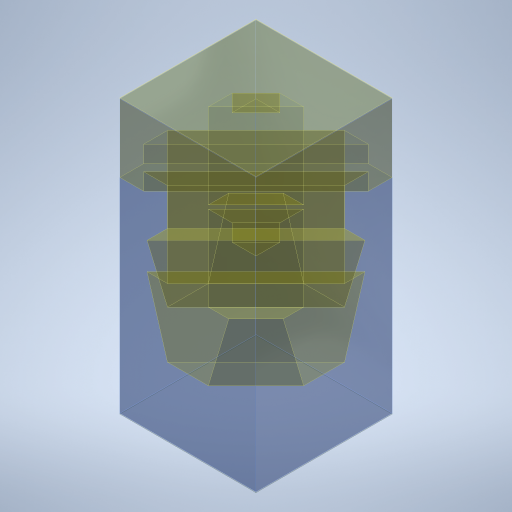
# Autodesk Inventor part: J1
Saved by Autodesk Inventor 2024 (Build 280153000, 153)
## iProperties
Created: 2013-03-22
Part Number: J1
Material: Generic
Document SubType Name: Modeling
Designer: User
Density: 1 g/cm^3
Appearance: Default
Author: User
Autodesk Inventor part; units mm, degrees
ref_plane "YZ Plane" through (0, 0, 0) normal (1, 0, 0) x (0, 1, 0)
ref_plane "XY Plane" through (0, 0, 0) normal (0, 0, 1) x (1, 0, 0)
ref_plane "Work Plane1" through (0, 180, -120) normal (0, 1, 0) x (-1, 0, 0)
sketch "Sketch3" plane through (0, 0, 0) normal (0, 0, 1) x (1, 0, 0)
  line L0 (-36, 180) -> (216, 180) projected
  line L1 (0, 0) -> (180, 0)
  line L2 (180, 0) -> (180, 180)
  line L3 (180, 180) -> (0, 180)
  line L4 (0, 180) -> (0, 0)
  dimension "d3" = 180
  constraints: 8 end point, 2 parallel, 2 perpendicular, 1 collinear, 1 horizontal
  measures "d3" distance of L3.end L1.start
extrude "Extrusion1" add sketch "Sketch3" along normal blind 360
ref_plane "Midlle" through (180, 180, 180) normal (0, 0, 1) x (1, 0, 0)
ref_plane "Work Plane2" through (180, 0, 0) normal (-0.7071068, -0.7071068, 0) x (0, 0, 1)
sketch "Sketch4" plane through (180, 0, 0) normal (-0.7071068, -0.7071068, 0) x (0, 0, 1)
  line L0 (360, 0) -> (0, 0) projected
  line L1 (0, 0) -> (0, 254.5584) projected
  line L2 (0, 254.5584) -> (360, 254.5584) projected
  line L3 (360, 254.5584) -> (360, 0) projected
  line L4 (0, 127.2792) -> (360, 127.2792) construction
  line L5 (270, 254.5584) -> (270, 232.2846)
  line L6 (270, 232.2846) -> (292.2739, 232.2846)
  line L7 (292.2739, 232.2846) -> (292.2739, 210.0107)
  line L8 (292.2739, 210.0107) -> (180, 210.0107)
  line L9 (180, 210.0107) -> (180, 229.1026)
  line L10 (180, 229.1026) -> (90, 210.0107)
  line L11 (90, 210.0107) -> (90, 171.8269)
  line L12 (90, 171.8269) -> (180, 152.7351)
  line L13 (180, 152.7351) -> (180, 171.8269)
  line L14 (180, 171.8269) -> (292.2739, 171.8269)
  line L15 (292.2739, 171.8269) -> (292.2739, 82.7315)
  line L16 (34.5859, 254.5584) -> (34.5859, 127.2792) construction
  line L17 (34.5859, 190.9188) -> (15.3416, 190.9188) construction
  line L18 (270, 22.2739) -> (292.2739, 22.2739)
  line L19 (292.2739, 22.2739) -> (292.2739, 44.5477)
  line L20 (292.2739, 44.5477) -> (180, 44.5477)
  line L21 (180, 44.5477) -> (180, 25.4558)
  line L22 (180, 25.4558) -> (90, 44.5477)
  line L23 (90, 44.5477) -> (90, 82.7315)
  line L24 (90, 82.7315) -> (180, 101.8234)
  line L25 (180, 101.8234) -> (180, 82.7315)
  line L26 (180, 82.7315) -> (292.2739, 82.7315)
  line L27 (270, 22.2739) -> (270, 0)
  line L28 (292.2739, 105.0054) -> (270, 105.0054)
  line L29 (270, 105.0054) -> (270, 149.5531)
  line L30 (270, 149.5531) -> (292.2739, 149.5531)
  line L31 (292.2739, 149.5531) -> (292.2739, 105.0054)
  line L32 (281.1369, 105.0054) -> (281.1369, 127.2792) construction
  point P0 (292.2739, 127.2792)
  dimension "d6" = 254.5584
  dimension "d9" = 360
  dimension "d25" = 127.2792
  dimension "d26" = 76.3675
  dimension "d27" = 19.0919
  dimension "d28" = 90
  dimension "d29" = 90
  dimension "d30" = 90
  constraints: 56 end point, 10 symmetric about line, 9 parallel, 7 perpendicular, 7 point on line, 4 midpoint, 3 equal length, 2 collinear, 1 horizontal, 3 other
  measures "d6" distance of L0.end L1.end
  measures "d9" distance of L1.end L2.end
  measures "d25" distance between parallel lines of L2 L4
  measures "d26" distance of L12.end L9.end
  measures "d27" distance of L8.end L9.end
  measures "d28" distance between parallel lines of L1 L11
  measures "d29" distance between parallel lines of L9 L11
  measures "d30" distance between parallel lines of L3 L5
extrude "Extrusion7" add sketch "Sketch4" against normal up to surface separate body contours L0 L27 L18 L19 L20 L21 L22 L23 L24 L25 L26 L15 L14 L13 L12 L11 L10 L9 L8 L7 L6 L5 L2 L3 | L28 L29 L30 L15 starts on plane at (0, 0, 0) facing (0, -1, 0) surface through (180, 180, 0) normal (0, 1, 0)
extrude "Extrusion8" cut sketch "Sketch3" along normal blind 360 keep common part bodies 2
extrude "Extrusion9" add sketch "Sketch4" against normal up to surface separate body contours L0 L1 L2 L5 L6 L7 L8 L9 L10 L11 L12 L13 L14 L15 L30 L29 L28 L26 L25 L24 L23 L22 L21 L20 L19 L18 L27 starts on plane at (0, 0, 0) facing (0, -1, 0) surface through (180, 180, 0) normal (0, 1, 0)
extrude "Extrusion10" cut sketch "Sketch3" along normal blind 360 keep common part bodies 3
move faces "Move Face3" translate (0, 0, 1) faces at (120, 60, 360) (120, 60, 360)
move faces "Move Face4" translate (0, 0, -1) faces at (120, 60, 0) (120, 60, 0)
equation "\"d4\" = 2 * d3"
equation "\"d26\" = 0.6 * d25"
equation "\"d27\" = 0.25 * d26"
equation "\"d28\" = 0.25 * d9"
equation "\"d29\" = d28"
equation "\"d30\" = d28"
equation "\"d31\" = 2 * d3"
equation "\"d33\" = 2 * d3"
equation "\"d35\" = 2 * d3"
equation "\"d37\" = 2 * d3"
